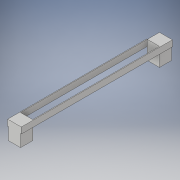
# Autodesk Inventor part: crossbeam
Saved by Autodesk Inventor 2018 (Build 220112000, 112)
## iProperties
Created: 2018-01-19
Part Number: crossbeam
Material: Generic
Document SubType Name: Modeling
Designer: S-2512711
Density: 1 g/cm^3
Appearance: Default
Author: S-2512711
Autodesk Inventor part; units mm, degrees
ref_plane "YZ Plane" through (0, 0, 0) normal (1, 0, 0) x (0, 1, 0)
ref_plane "XZ Plane" through (0, 0, 0) normal (0, 1, 0) x (-1, 0, 0)
ref_plane "XY Plane" through (0, 0, 0) normal (0, 0, 1) x (1, 0, 0)
sketch "Sketch1" plane through (0, 0, 0) normal (0, 1, 0) x (-1, 0, 0)
  line L0 (50.8, 341.3125) -> (0, 341.3125)
  line L1 (0, 341.3125) -> (0, 290.5125)
  line L2 (0, 290.5125) -> (50.8, 290.5125)
  line L3 (50.8, 290.5125) -> (50.8, 341.3125)
  line L4 (50.8, -290.5125) -> (0, -290.5125)
  line L5 (0, -290.5125) -> (0, -239.7125)
  line L6 (0, -239.7125) -> (50.8, -239.7125)
  line L7 (50.8, -239.7125) -> (50.8, -290.5125)
  line L8 (0, 0) -> (-42.6013, 0)
  dimension "d0" = 50.8
  dimension "d10" = 530.225
  constraints: 18 end point, 4 parallel, 4 perpendicular, 3 horizontal, 2 collinear, 1 point on line, 1 other
  measures "d0" distance of L2.end L0.start
  measures "d10" distance between parallel lines of L6 L2
extrude "Extrusion1" add sketch "Sketch1" along normal blind 76.2
sketch "Sketch2" plane through (0, 0, 341.3125) normal (1, 0, 0) x (0, 0, -1)
  line L0 (0, 76.2) -> (50.8, 76.2) projected
  line L1 (631.825, 0) -> (631.825, 76.2) projected
  line L2 (0, 76.2) -> (631.825, 76.2)
  line L3 (631.825, 76.2) -> (631.825, 50.8)
  line L4 (631.825, 50.8) -> (0, 50.8)
  line L5 (0, 50.8) -> (0, 76.2)
  point P0 (341.3125, 0)
  dimension "d4" = 25.4
  constraints: 8 end point, 2 parallel, 1 horizontal, 1 perpendicular, 1 point on line
  measures "d4" distance between parallel lines of L2 L4
extrude "Extrusion2" add sketch "Sketch2" along normal blind 3.175
sketch "Sketch3" plane through (-50.8, 0, 290.5125) normal (-1, 0, 0) x (0, 0, 1)
  line L0 (50.8, 76.2) -> (-530.225, 76.2)
  line L1 (-530.225, 76.2) -> (-530.225, 50.8)
  line L2 (-530.225, 50.8) -> (50.8, 50.8)
  line L3 (50.8, 50.8) -> (50.8, 76.2)
  line L4 (-530.225, 50.8) -> (0, 50.8) projected
  point P0 (-290.5125, 0)
  constraints: 8 end point, 2 parallel, 1 collinear, 1 horizontal, 1 perpendicular
extrude "Extrusion3" add sketch "Sketch3" along normal blind 3.175
body "Solid1"
